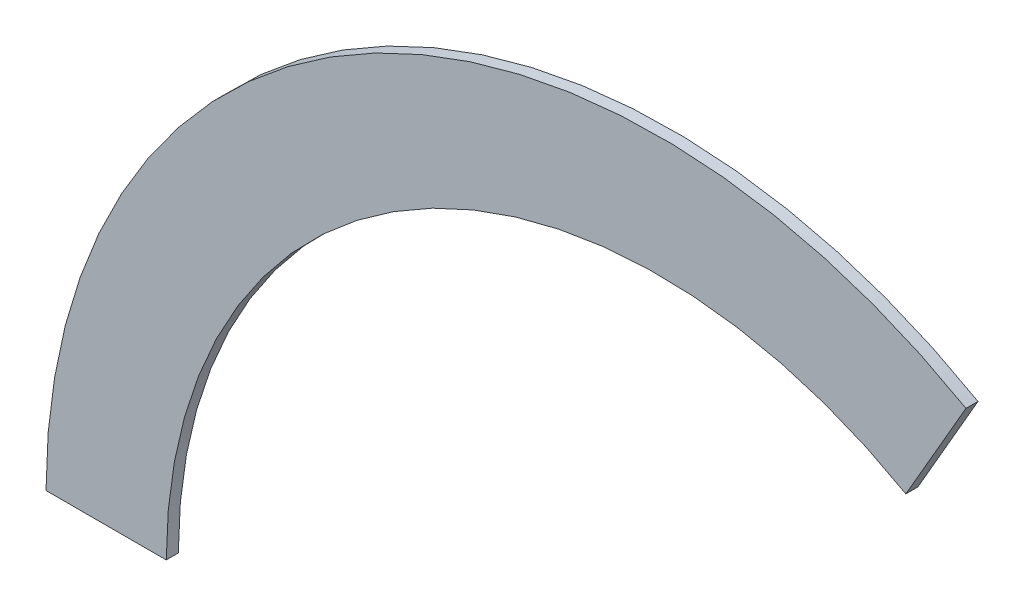
# Autodesk Inventor part: BSH 083 barrel amplifier
Saved by Autodesk Inventor 2025 (Build 290162010, 162A)
## iProperties
Created: 2024-08-04
Part Number: BSH 083 barrel amplifier
Material: Stainless Steel
Document SubType Name: Sheet Metal
Designer: pokla
Density: 8 g/cm^3
Sheet Metal Rule: AISI304 2mm Die16
Appearance: Default
Author: pokla
Autodesk Inventor part; units mm, degrees
ref_plane "YZ Plane" through (0, 0, 0) normal (1, 0, 0) x (0, 1, 0)
ref_plane "XZ Plane" through (0, 0, 0) normal (0, 1, 0) x (-1, 0, 0)
ref_plane "XY Plane" through (0, 0, 0) normal (0, 0, 1) x (1, 0, 0)
sketch "Sketch1" plane through (0, 0, 0) normal (0, 1, 0) x (-1, 0, 0)
  line L0 (410, 5) -> (510, 5)
  line L1 (510, 5) -> (510, -5)
  line L2 (510, -5) -> (410, -5)
  line L3 (410, -5) -> (410, 5)
  line L4 (0, 85.4801) -> (0, -85.4801)
  point P0 (0, 0)
  point P1 (0, 0)
  point P2 (410, 0)
  dimension "d0" = 100
  dimension "d1" = 410
  dimension "d2" = 10
  constraints: 10 end point, 2 midpoint, 2 parallel, 1 coincident, 1 horizontal, 1 horizontal alignment, 1 perpendicular, 1 vertical
  measures "d0" distance of L0.start L0.end
  measures "d1" distance of point (410, 0) point (0, 0)
  measures "d2" distance between parallel lines of L2 L0
revolve "Revolution1" add sketch "Sketch1" angle 120 about axis through (0, 0, 85.4801) along (0, 0, -1)
equation "\"BendReliefWidth\" = Thickness"
equation "\"BendReliefDepth\" = 0.5 * Thickness"
equation "\"CornerReliefSize\" = 4 * Thickness"
equation "\"MinimumRemnant\" = 2 * Thickness"
equation "\"TransitionRadius\" = BendRadius"
equation "\"JacobiRadiusSize\" = BendRadius"
equation "\"GapSize\" = Thickness"
equation "\"Thickness\" = 2"
equation "\"BendRadius\" = 2.75"
body "Solid1"
